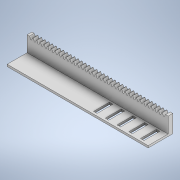
# Autodesk Inventor part: Rack
Saved by Autodesk Inventor 2020 (Build 240168000, 168)
## iProperties
Created: 2020-11-24
Part Number: Rack
Material: Generic
Document SubType Name: Modeling
Designer: shaun
Density: 1 g/cm^3
Appearance: Default
Author: shaun
Autodesk Inventor part; units mm, degrees
ref_plane "YZ Plane" through (0, 0, 0) normal (1, 0, 0) x (0, 1, 0)
ref_plane "XZ Plane" through (0, 0, 0) normal (0, 1, 0) x (-1, 0, 0)
ref_plane "XY Plane" through (0, 0, 0) normal (0, 0, 1) x (1, 0, 0)
sketch "Sketch1" plane through (0, 0, 0) normal (0, 0, 1) x (1, 0, 0)
  spline S0 degree 3 poles (-1.3621, 13.5316) (-1.3292, 13.4857) (-1.2634, 13.394) (-1.1694, 13.2531) (-1.0789, 13.11) (-0.9926, 12.9642) (-0.9108, 12.816) (-0.8338, 12.6651) (-0.7622, 12.5116) (-0.6965, 12.3555) (-0.6377, 12.1967) (-0.5868, 12.0351) (-0.5531, 11.898) (-0.533, 11.7869) (-0.5104, 11.7051) (-0.4797, 11.6261) (-0.4449, 11.5644) (-0.4127, 11.518) (-0.3847, 11.4862) (-0.355, 11.4559) (-0.3216, 11.4298) (-0.2867, 11.4058) (-0.2487, 11.3868) (-0.2098, 11.37) (-0.1686, 11.36) (-0.1271, 11.3512) (-0.0705, 11.3492) (0, 11.3505) (0.0705, 11.3492) (0.1271, 11.3512) (0.1686, 11.36) (0.2098, 11.37) (0.2487, 11.3868) (0.2867, 11.4058) (0.3216, 11.4298) (0.355, 11.4559) (0.3847, 11.4862) (0.4127, 11.518) (0.4449, 11.5644) (0.4797, 11.6261) (0.5104, 11.7051) (0.533, 11.7869) (0.5531, 11.898) (0.5868, 12.0351) (0.6377, 12.1967) (0.6965, 12.3555) (0.7622, 12.5116) (0.8338, 12.6651) (0.9108, 12.816) (0.9926, 12.9642) (1.0789, 13.11) (1.1694, 13.2531) (1.2634, 13.394) (1.3292, 13.4857) (1.3621, 13.5316) knots 0 0 0 0 0.016933 0.033866 0.0508 0.067733 0.084666 0.101599 0.118531 0.135464 0.152396 0.169328 0.186257 0.194723 0.203188 0.211652 0.220111 0.224346 0.228579 0.232811 0.237045 0.241276 0.245509 0.249742 0.253974 0.258206 0.262439 0.270905 0.279372 0.283605 0.287836 0.292069 0.296302 0.300535 0.304766 0.309 0.313231 0.317465 0.3217 0.330159 0.338623 0.347088 0.355554 0.372483 0.389415 0.406347 0.423279 0.440212 0.457145 0.474078 0.491011 0.507944 0.524878 0.541811 0.541811 0.541811 0.541811
  circle A0 centre (0, 0) radius 11.35 construction
  circle A1 centre (0, 0) radius 11.7462 construction
  circle A2 centre (0, 0) radius 12.5 construction
  line L0 (-1.3621, 13.5316) -> (1.3621, 13.5316)
  point P0 (-1.2642, 13.3934)
  point P1 (-1.17, 13.2527)
  point P2 (-1.0796, 13.1095)
  point P3 (-0.9933, 12.9638)
  point P4 (-0.9116, 12.8155)
  point P5 (-0.8347, 12.6647)
  point P6 (-0.7632, 12.5112)
  point P7 (-0.6976, 12.3551)
  point P8 (-0.639, 12.1962)
  point P9 (-0.5886, 12.0346)
  point P10 (-0.5486, 11.8701)
  point P11 (-0.5317, 11.7871)
  point P12 (-0.509, 11.7056)
  point P13 (-0.4778, 11.6269)
  point P14 (-0.4365, 11.5531)
  point P15 (-0.4121, 11.5185)
  point P16 (-0.3844, 11.4864)
  point P17 (-0.3544, 11.4566)
  point P18 (-0.3214, 11.4301)
  point P19 (-0.2862, 11.4066)
  point P20 (-0.2486, 11.3872)
  point P21 (-0.2094, 11.3711)
  point P22 (-0.1685, 11.3602)
  point P23 (-0.1269, 11.3524)
  point P24 (-0.0847, 11.35)
  point P25 (0, 11.35)
  point P26 (0.0847, 11.35)
  point P27 (0.1269, 11.3524)
  point P28 (0.1685, 11.3602)
  point P29 (0.2094, 11.3711)
  point P30 (0.2486, 11.3872)
  point P31 (0.2862, 11.4066)
  point P32 (0.3214, 11.4301)
  point P33 (0.3544, 11.4566)
  point P34 (0.3844, 11.4864)
  point P35 (0.4121, 11.5185)
  point P36 (0.4365, 11.5531)
  point P37 (0.4778, 11.6269)
  point P38 (0.509, 11.7056)
  point P39 (0.5317, 11.7871)
  point P40 (0.5486, 11.8701)
  point P41 (0.5886, 12.0346)
  point P42 (0.639, 12.1962)
  point P43 (0.6976, 12.3551)
  point P44 (0.7632, 12.5112)
  point P45 (0.8347, 12.6647)
  point P46 (0.9116, 12.8155)
  point P47 (0.9933, 12.9638)
  point P48 (1.0796, 13.1095)
  point P49 (1.17, 13.2527)
  point P50 (1.2642, 13.3934)
  constraints: 3 centre point, 2 end point, 1 horizontal, 110 other
sketch "Sketch2" plane through (0, 0, 0) normal (0, 0, 1) x (1, 0, 0)
  line L0 (-3.3621, 13.5316) -> (116.6379, 13.5316)
  line L1 (116.6379, 13.5316) -> (116.6379, 9.5316)
  line L2 (116.6379, 9.5316) -> (-3.3621, 9.5316)
  line L3 (-3.3621, 9.5316) -> (-3.3621, 13.5316)
  line L4 (-1.3621, 13.5316) -> (1.3621, 13.5316) projected
  point P0 (0, 0)
  point P1 (0, 13.5316)
  dimension "d7" = 120
  dimension "d8" = 4
  dimension "d9" = 2
  constraints: 8 end point, 2 parallel, 1 horizontal, 1 midpoint, 1 perpendicular, 1 point on line
  measures "d7" distance between parallel lines of L1 L3
  measures "d8" distance between parallel lines of L2 L0
  measures "d9" distance from line of L3 L4.start
extrude "Extrusion3" add sketch "Sketch2" against normal blind 4
extrude "Extrusion4" cut sketch "Sketch1" against normal blind 4
pattern_linear "Rectangular Pattern1" count 37 spacing 3.1416 along (1, 0, 0) of "Extrusion4"
sketch "Sketch3" plane through (-3.3621, 9.5316, 0) normal (-1, 0, 0) x (0, 0, 1)
  line L0 (0, 0) -> (-4, 0) projected
  line L1 (0, 0) -> (0, -11)
  line L2 (0, -11) -> (-4, -11)
  line L3 (-4, -11) -> (-4, 0)
  line L4 (-4, 0) -> (0, 0)
  line L5 (0, -11) -> (17, -11)
  line L6 (17, -11) -> (17, -9.25)
  line L7 (17, -9.25) -> (0, -9.25)
  point P0 (0, -9.5316)
  dimension "d17" = 11
  dimension "d18" = 17
  dimension "d19" = 1.75
  constraints: 14 end point, 4 perpendicular, 1 collinear, 1 horizontal, 1 point on line, 1 vertical
  measures "d17" distance of L0.start L1.end
  measures "d18" distance of L1.end L5.end
  measures "d19" distance of L5.end L6.end
extrude "Extrusion5" add sketch "Sketch3" against normal blind 120
sketch "Sketch4" plane through (-3.3621, 0.2816, 17) normal (0, 1, 0) x (1, 0, 0)
  line L0 (120, 0) -> (120, 21) projected
  line L1 (114.5251, 15.4999) -> (111.5251, 15.4999)
  line L2 (111.5251, 15.4999) -> (111.5251, 2)
  line L3 (111.5251, 2) -> (114.5251, 2)
  line L4 (114.5251, 2) -> (114.5251, 15.4999)
  line L5 (94.5251, 2) -> (94.5251, 15.4999)
  line L6 (91.5251, 15.4999) -> (91.5251, 2)
  line L7 (91.5251, 2) -> (94.5251, 2)
  line L8 (94.5251, 15.4999) -> (91.5251, 15.4999)
  line L9 (74.5251, 2) -> (74.5251, 15.4999)
  line L10 (71.5251, 15.4999) -> (71.5251, 2)
  line L11 (71.5251, 2) -> (74.5251, 2)
  line L12 (74.5251, 15.4999) -> (71.5251, 15.4999)
  line L13 (54.5251, 2) -> (54.5251, 15.4999)
  line L14 (51.5251, 15.4999) -> (51.5251, 2)
  line L15 (51.5251, 2) -> (54.5251, 2)
  line L16 (54.5251, 15.4999) -> (51.5251, 15.4999)
  line L17 (34.5251, 2) -> (34.5251, 15.4999)
  line L18 (31.5251, 15.4999) -> (31.5251, 2)
  line L19 (31.5251, 2) -> (34.5251, 2)
  line L20 (34.5251, 15.4999) -> (31.5251, 15.4999)
  line L21 (14.5251, 2) -> (14.5251, 15.4999)
  line L22 (11.5251, 15.4999) -> (11.5251, 2)
  line L23 (11.5251, 2) -> (14.5251, 2)
  line L24 (14.5251, 15.4999) -> (11.5251, 15.4999)
  line L25 (101.5251, 15.4999) -> (101.5251, 2)
  line L26 (104.5251, 2) -> (104.5251, 15.4999)
  line L27 (104.5251, 15.4999) -> (101.5251, 15.4999)
  line L28 (101.5251, 2) -> (104.5251, 2)
  line L29 (91.5251, 15.4999) -> (91.5251, 2)
  line L30 (94.5251, 2) -> (94.5251, 15.4999)
  line L31 (94.5251, 15.4999) -> (91.5251, 15.4999)
  line L32 (91.5251, 2) -> (94.5251, 2)
  line L33 (81.5251, 15.4999) -> (81.5251, 2)
  line L34 (84.5251, 2) -> (84.5251, 15.4999)
  line L35 (84.5251, 15.4999) -> (81.5251, 15.4999)
  line L36 (81.5251, 2) -> (84.5251, 2)
  line L37 (71.5251, 15.4999) -> (71.5251, 2)
  line L38 (74.5251, 2) -> (74.5251, 15.4999)
  line L39 (74.5251, 15.4999) -> (71.5251, 15.4999)
  line L40 (71.5251, 2) -> (74.5251, 2)
  point P0 (3.3621, 17)
  point P1 (120, 2)
  point P2 (95.2889, 15.4999)
  point P3 (92.2889, 2)
  point P4 (72.2889, 2)
  point P5 (75.2889, 15.4999)
  point P6 (52.2889, 2)
  point P7 (55.2889, 15.4999)
  point P8 (32.2889, 2)
  point P9 (35.2889, 15.4999)
  point P10 (12.2889, 2)
  point P11 (15.2889, 15.4999)
  point P12 (-7.7111, 2)
  point P13 (-4.7111, 15.4999)
  point P14 (85.2889, 15.4999)
  point P15 (82.2889, 2)
  point P16 (75.2889, 15.4999)
  point P17 (72.2889, 2)
  point P18 (65.2889, 15.4999)
  point P19 (62.2889, 2)
  point P20 (55.2889, 15.4999)
  point P21 (52.2889, 2)
  dimension "d22" = 2
  dimension "d24" = 3
  dimension "d27" = 20
  dimension "d36" = 10
  constraints: 80 end point, 21 point on line, 3 horizontal, 2 collinear, 2 parallel, 1 perpendicular, 88 other
  measures "d22" distance of L0.start point (120, 2)
  measures "d24" distance between parallel lines of L2 L4
  measures "d27" distance of L3.end L5.start
  measures "d36" distance of L1.end L25.start
extrude "Extrusion6" cut sketch "Sketch4" against normal blind 120 contours L4 L3 L2 L1 | L7 L6 L8 L5 | L11 L10 L12 L9 | L27 L26 L28 L25 | L35 L34 L36 L33
equation "\"Module\" = 1"
equation "\"PressureAngle\" = 20deg"
equation "\"UnitProfileClearance\" = 0.25"
equation "\"UnitRoundRadius\" = 0.35"
equation "\"HeadDiameter\" = 27.2"
equation "\"RootDiameter\" = 22.7"
equation "\"BaseDiameter\" = 23.49232"
equation "\"PitchDiameter\" = 25"
equation "\"FaceWidth\" = 3"
equation "\"HelixAngle\" = 0"
equation "\"UnitCorrection\" = 0.1"
equation "\"UnitAddendumModification\" = 0"
equation "\"CircularPitch\" = 3.141593"
equation "\"UnitBacklashShift\" = 0"
equation "\"TotalToolShift\" = 0.1"
equation "\"IsInternal\" = 0"
body "Solid2"
